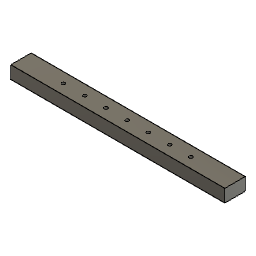
Stencil Drill Fixture v2 (Autodesk Fusion 360 design; units mm, degrees)
Autodesk Fusion 360 part; units mm, degrees
sketch "Sketch1" plane through (0, 0, 0) normal (0, 1, 0) x (1, 0, 0)
  line L0 (-125, 10) -> (125, 10) construction
  line L1 (125, 10) -> (125, -10) construction
  line L2 (125, -10) -> (-125, -10) construction
  line L3 (-125, -10) -> (-125, 10) construction
  line L4 (-125, 10) -> (125, -10) construction
  line L5 (125, 10) -> (-125, -10) construction
  line L6 (-125.1, 10.05) -> (125, 10.05)
  line L7 (125, -10.05) -> (-125.1, -10.05)
  line L8 (-125.1, -10.05) -> (-125.1, 10.05)
  line L9 (-125, 12) -> (125, 12)
  line L10 (125, 12) -> (125, -12)
  line L11 (125, -12) -> (-125, -12)
  line L12 (-125, -12) -> (-125, 12)
  line L13 (-125, 12) -> (125, -12) construction
  line L14 (125, 12) -> (-125, -12) construction
  line L15 (125, -12) -> (127, -12)
  line L16 (127, -12) -> (127, 12)
  line L17 (127, 12) -> (125, 12)
  line L18 (125, 12) -> (125, -12)
  circle A0 centre (0, 0) radius 2
  circle A1 centre (-75, 0) radius 2
  circle A2 centre (-50, 0) radius 2
  circle A3 centre (-25, 0) radius 2
  circle A4 centre (25, 0) radius 2
  circle A5 centre (50, 0) radius 2
  circle A6 centre (75, 0) radius 2
  dimension "d1" = 250
  dimension "d2" = 20
  dimension "d4" = 250
  dimension "d5" = 24
  dimension "d6" = 2
  dimension "d7" = 4
  dimension "d10" = 25
  dimension "d11" = 0
  constraint horizontal L0
  constraint perpendicular L0 L1
  constraint parallel L0 L2
  constraint parallel L1 L3
  constraint coincident L4 A0.centre
  constraint coincident L5 A0.centre
  constraint coincident A0.centre origin
  constraint horizontal L9
  constraint perpendicular L9 L10
  constraint parallel L9 L11
  constraint parallel L10 L12
  constraint coincident L13 A0.centre
  constraint coincident L14 A0.centre
  constraint horizontal L15
  constraint vertical L16
  constraint horizontal L17
  constraint vertical L18
  constraint coincident L9.end L10.start
  constraint coincident L6.end L18
  constraint coincident L7.start L10
  measures "d1" distance of L1.end L2.end
  measures "d2" distance of L0.end L1.end
  measures "d4" distance of L10.end L11.end
  measures "d5" distance of L9.end L10.end
  measures "d6" distance of L10.end L15.end
  measures "d7" diameter of A0
extrude "Extrude1" add sketch "Sketch1" along normal blind 10 contours L6 L9 L10 L12 L18 | L6 L7 L10 L12 L18 | L10 L15 L16 L17 L18 | L7 L10 L11 L12 L18
extrude "Extrude2" add sketch "Sketch1" against normal blind 5 contours L6 L9 L10 L12 L18 | L10 L15 L16 L17 L18 | L7 L10 L11 L12 L18
named bodies: "Stencil - Drill Fixture"
